Scheibe fürSG90_v1 (Autodesk Fusion 360 design; units mm, degrees)
Autodesk Fusion 360 part; units mm, degrees
cylinder "Grundkörper Zylinder1" add diameter 9 height 10 placed x (1, 0, 0) y (0, 0, -1) z (0, 1, 0) at (0, 0, 0)
cylinder "Grundkörper Zylinder2" cut diameter 4.4 height -3.2 placed x (1, 0, 0) y (0, 0, -1) z (0, 1, 0) at (0, 10, 0)
cylinder "Grundkörper Zylinder3" cut diameter 2.6 height -21 placed x (1, 0, 0) y (0, 0, -1) z (0, 1, 0) at (0, 6.8, 0)
cylinder "Grundkörper Zylinder4" cut diameter 5 height -6 placed x (1, 0, 0) y (0, 0, 1) z (0, -1, 0) at (0, 0, 0)
sketch "Skizze5" plane through (0, 0, 0) normal (0, -1, 0) x (1, 0, 0)
  circle A0 centre (0, 0) radius 2.5
  circle A1 centre (0, 0) radius 4.5
  circle A2 centre (0, 0) radius 9
  circle A3 centre (0, 0) radius 6.75
  circle A4 centre (0, 6.75) radius 1
  circle A5 centre (3.375, 5.8457) radius 1
  circle A6 centre (5.8457, 3.375) radius 1
  circle A7 centre (6.75, 0) radius 1
  circle A8 centre (5.8457, -3.375) radius 1
  circle A9 centre (3.375, -5.8457) radius 1
  circle A10 centre (0, -6.75) radius 1
  circle A11 centre (-3.375, -5.8457) radius 1
  circle A12 centre (-3.375, 5.8457) radius 1
  circle A13 centre (-5.8457, 3.375) radius 1
  circle A14 centre (-6.75, 0) radius 1
  circle A15 centre (-5.8457, -3.375) radius 1
  dimension "d9" = 18
  dimension "d10" = 13.5
  dimension "d11" = 2
  dimension "d12" = 2
  dimension "d13" = 2
  dimension "d14" = 2
  dimension "d15" = 2
  dimension "d16" = 2
  dimension "d17" = 2
  dimension "d18" = 2
  dimension "d19" = 2
  dimension "d20" = 2
  dimension "d21" = 2
  dimension "d22" = 2
  constraint coincident A0.centre A1.centre
  constraint coincident A3 A4.centre
  measures "d9" diameter of A2
  measures "d10" diameter of A3
  measures "d11" diameter of A4
  measures "d12" diameter of A5
  measures "d13" diameter of A6
  measures "d14" diameter of A7
  measures "d15" diameter of A8
  measures "d16" diameter of A9
  measures "d17" diameter of A10
  measures "d18" diameter of A11
  measures "d19" diameter of A15
  measures "d20" diameter of A14
  measures "d21" diameter of A13
  measures "d22" diameter of A12
extrude "Extrusion1" add sketch "Skizze5" against normal blind 4 contours A2 | A3 A4 A5 A6 A7 A8 A9 A10 A11 A12 A13 A14 A15
